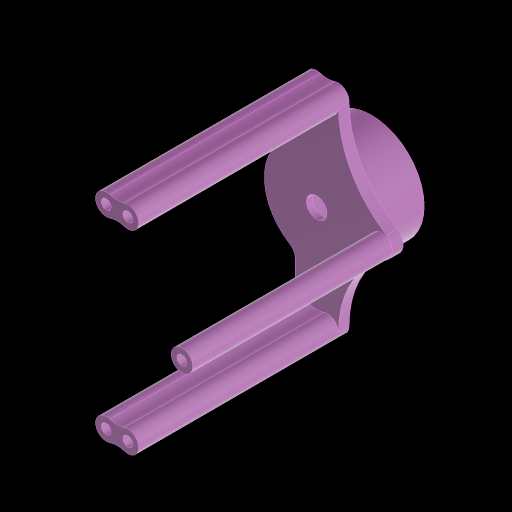
# Autodesk Inventor part: MotorMountShuffler Pod
Saved by Autodesk Inventor 2023 (Build 270158000, 158)
## iProperties
Created: 2022-03-05
Part Number: MotorMountShuffler Pod
Material: Custom TPU
Document SubType Name: Modeling
Designer: tandu
Density: 1.21 g/cm^3
Appearance: Smooth - Purple
TopStandoffOffset1: 0.75000000 in
Author: tandu
Autodesk Inventor part; units mm, degrees
ref_plane "YZ Plane" through (0, 0, 0) normal (1, 0, 0) x (0, 1, 0)
ref_plane "XZ Plane" through (0, 0, 0) normal (0, 1, 0) x (-1, 0, 0)
ref_plane "XY Plane" through (0, 0, 0) normal (0, 0, 1) x (1, 0, 0)
sketch "Sketch1" plane through (0, 0, 0) normal (0, 0, 1) x (1, 0, 0)
  circle A0 centre (0, 0) radius 12 construction
  circle A1 centre (0, 0) radius 3.048
  circle A2 centre (0, 0) radius 12.254
  circle A3 centre (0, 0) radius 15.429
  line L0 (6.35, 31.75) -> (-6.35, 31.75)
  line L1 (-6.35, 31.75) -> (-6.35, -31.75)
  line L2 (-6.35, -31.75) -> (6.35, -31.75)
  line L3 (6.35, -31.75) -> (6.35, 31.75)
  line L4 (6.35, 31.75) -> (-6.35, -31.75) construction
  line L5 (-6.35, 31.75) -> (6.35, -31.75) construction
  circle A4 centre (19.05, 0) radius 3.175
  circle A5 centre (3.175, -28.575) radius 3.175
  circle A6 centre (-3.175, -28.575) radius 3.175
  circle A7 centre (3.175, 28.575) radius 3.175
  circle A8 centre (-3.175, 28.575) radius 3.175
  circle A9 centre (-19.05, 0) radius 3.175
  line L6 (0, 0) -> (-19.05, 0) construction
  line L7 (0, 0) -> (19.05, 0) construction
  arc A10 (20.4611, -3.175) -> (20.4611, 3.175) centre (18.4856, 0) ccw
  arc A11 (20.4611, -3.175) -> (6.35, -28.575) centre (36.2656, -28.575) ccw
  arc A12 (6.35, 28.575) -> (20.4611, 3.175) centre (36.2656, 28.575) ccw
  line L8 (0, -31.75) -> (0, 31.75) construction
  arc A13 (-20.4611, 3.175) -> (-20.4611, -3.175) centre (-18.4856, 0) ccw
  arc A14 (-6.35, -28.575) -> (-20.4611, -3.175) centre (-36.2656, -28.575) ccw
  arc A15 (-20.4611, 3.175) -> (-6.35, 28.575) centre (-36.2656, 28.575) ccw
  circle A16 centre (0, 0) radius 7
  arc A17 (-2.1167, 31.5684) -> (2.1167, 31.5684) centre (0, 37.5553) ccw
  arc A18 (2.1167, -31.5684) -> (-2.1167, -31.5684) centre (0, -37.5553) ccw
  arc A19 (2.1167, 25.5816) -> (-2.1167, 25.5816) centre (0, 19.5947) ccw
  arc A20 (-2.1167, -25.5816) -> (2.1167, -25.5816) centre (0, -19.5947) ccw
  point P0 (-6.35, 14.0617)
  point P1 (6.35, 14.0617)
  point P2 (6.35, -14.0617)
  point P3 (-6.35, -14.0617)
  point P4 (-6.35, -28.575)
  point P5 (-3.175, -31.75)
  point P6 (3.175, -31.75)
  point P7 (6.35, -28.575)
  point P8 (6.35, 28.575)
  point P9 (3.175, 31.75)
  point P10 (-3.175, 31.75)
  point P11 (-6.35, 28.575)
  point P12 (-14.0861, -6.2957)
  point P13 (-19.05, -3.175)
  point P14 (-19.05, 3.175)
  point P15 (-14.0861, 6.2957)
  point P16 (19.05, 3.175)
  point P17 (19.05, -3.175)
  point P18 (-6.35, 28.575)
  point P19 (-22.225, 0)
  point P20 (-6.35, -28.575)
  point P21 (22.225, 0)
  point P22 (2.1167, -31.5684)
  point P23 (2.1167, -25.5816)
  point P24 (-2.1167, -25.5816)
  point P25 (0, -28.575)
  point P26 (0, 28.575)
  dimension "d0" = 24
  dimension "d1" = 6.096
  dimension "d2" = 0.254
  dimension "d3" = 3.175
  dimension "d6" = 12.7
  dimension "d7" = 63.5
  dimension "d10" = 6.35
  dimension "d11" = 6.35
  dimension "d15" = 19.05
  dimension "d19" = 3.175
  dimension "d26" = 14
  dimension "d29" = 6.35
  constraints: 30 point on circle, 21 centre point, 18 end point, 18 tangent, 13 symmetric about line, 5 equal radius, 5 midpoint, 3 coincident, 3 horizontal, 2 horizontal alignment, 2 parallel, 2 point on line, 1 collinear, 1 perpendicular, 1 vertical alignment, 5 other
  measures "d0" diameter of A0
  measures "d1" diameter of A1
  measures "d2" radial gap between concentric circles of A0 A2
  measures "d3" radial gap between concentric circles of A2 A3
  measures "d6" distance of L2.end L1.end
  measures "d7" distance of L1.end L0.end
  measures "d10" diameter of A4
  measures "d11" diameter of A5
  measures "d15" distance of L6.start L7.end
  measures "d19" vertical distance of L7.end A10.start
  measures "d26" diameter of A16
  measures "d29" radius of A17
extrude "CircularMotorMount" add sketch "Sketch1" against normal blind 13 contours A2 L3 A3 | A2 L1 A3 L3 | L3 A3 L1 A2 | A2 L1 A3
extrude "Plate" add sketch "Sketch1" along normal blind 3.175 contours A2 L3 A16 | A2 L3 A3 | L3 A16 L1 A2 | A2 L1 A3 L3 | L3 A3 L1 A2 | A2 L1 A16 L3 | L1 A16 A2 | A2 L1 A3 | A16 L3 | L3 A16 L1 | A4 | L3 A12 A10 A11 A3 | A3 L1 A8 A19 A7 L3 | L3 A5 A20 A6 L1 A3 | L1 A16 | A7 | A5 | A8 | A19 A8 A7 | A6 | A5 A6 A20 | A8 A17 A7 | A5 A18 A6
extrude "StandOffLikeThings" add sketch "Sketch1" along normal blind 58.674 from surface at 3.175 contours A4 | A7 | A5 | A8 | A19 A8 A7 | A6 | A5 A6 A20 | A8 A17 A7 | A5 A18 A6
fillet "Fillet1" radius 3.175 2 edges at (-6.35, 14.0617, 1.5875) (-6.35, -14.0617, 1.5875)
sketch "Sketch2" plane through (-3.175, 28.575, 61.849) normal (0, 0, 1) x (0, -1, 0)
  arc A0 (-2.9934, 1.0583) -> (2.9934, 1.0583) centre (0, 0) ccw projected
  arc A1 (2.9934, 5.2917) -> (-2.9934, 5.2917) centre (0, 6.35) ccw projected
  arc A2 (54.1566, 1.0583) -> (60.1434, 1.0583) centre (57.15, 0) ccw projected
  arc A3 (60.1434, 5.2917) -> (54.1566, 5.2917) centre (57.15, 6.35) ccw projected
  circle A4 centre (57.15, 0) radius 1.4732
  circle A5 centre (57.15, 6.35) radius 1.4732
  circle A6 centre (0, 0) radius 1.4732
  circle A7 centre (0, 6.35) radius 1.4732
  circle A8 centre (28.575, 22.225) radius 3.175 projected
  circle A9 centre (28.575, 22.225) radius 1.4732
  point P0 (28.575, 3.175)
  dimension "d21" = 2.9464
  constraints: 5 centre point, 5 coincident, 4 equal radius
  measures "d21" diameter of A4
extrude "Extrusion4" cut sketch "Sketch2" against normal blind 9.525 contours A4 | A5 | A6 | A7 | A9
extrude "Extrusion5" [suppressed]
extrude "MotorExtraPocketing" cut sketch "Sketch1" along normal blind 1.5 contours A1 | A16 L3 | L3 A16 L1 | L1 A16
equation "\"d7\" = ShufflerPodWidth"
equation "\"d15\" = TopStandoffOffset1"
equation "\"TopStandoffOffset1\" = TopStandoffOffset"
equation "\"ShufflerPodWidth\" = 63.5"
equation "\"TopStandoffOffset\" = 19.05"
body "Solid1"
